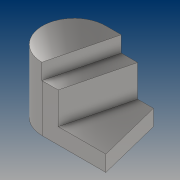
# Autodesk Inventor part: 6
Saved by Autodesk Inventor 2020.2 (Build 242310000, 310)
## iProperties
Created: 2020-09-17
Part Number: 6
Material: 鋼、碳鋼
Document SubType Name: Modeling
Designer: user
Density: 7.85 g/cm^3
Appearance: 半拋光
Mass: 416.126 g
Surface Area: 96.1298 cm^2
Volume: 53.0096 cm^3
Author: user
Autodesk Inventor part; units mm, degrees
ref_plane "YZ Plane" through (0, 0, 0) normal (1, 0, 0) x (0, 1, 0)
ref_plane "XZ Plane" through (0, 0, 0) normal (0, 1, 0) x (-1, 0, 0)
ref_plane "XY Plane" through (0, 0, 0) normal (0, 0, 1) x (1, 0, 0)
sketch "草圖1" plane through (0, 0, 0) normal (0, 1, 0) x (-1, 0, 0)
  circle A0 centre (0, 0) radius 20
  line L0 (0, -20) -> (-40, -20)
  line L1 (-40, -20) -> (-40, 20)
  line L2 (-40, 20) -> (0, 20)
  line L3 (0, 20) -> (0, -20)
  point P0 (0, 20)
  dimension "d0" = 40
  dimension "d1" = 40
  constraints: 8 end point, 3 horizontal, 2 parallel, 1 coincident, 1 perpendicular, 3 other
  measures "d1" distance of L0.start L0.end
extrude "擠出1" add sketch "草圖1" along normal blind 40
sketch "草圖2" plane through (0, 40, 0) normal (0, 1, 0) x (1, 0, 0)
  line L0 (0, 20) -> (40, 20) projected
  line L1 (40, 20) -> (40, -20) projected
  line L2 (40, -20) -> (0, -20) projected
  arc A0 (0, 20) -> (0, -20) centre (0, 0) ccw projected
  line L3 (0, -20) -> (40, -20) projected
  line L4 (40, -20) -> (30, 20)
  dimension "d4" = 10
  constraints: 2 end point, 1 point on line
  measures "d4" distance from line of L4.end L1
extrude "擠出2" cut sketch "草圖2" against normal through all contours L0 L1 L4
sketch "草圖3" plane through (0, 40, 0) normal (0, 1, 0) x (1, 0, 0)
  line L0 (30, 20) -> (0, 20) projected
  line L1 (20, 20) -> (10, -20)
  line L2 (0, -20) -> (40, -20) projected
  line L3 (30, 20) -> (40, -20) projected
  line L4 (40, -20) -> (0, -20) projected
  arc A0 (0, 20) -> (0, -20) centre (0, 0) ccw projected
  line L5 (0, 20) -> (30, 20) projected
  dimension "d7" = 10
  dimension "d8" = 30
  constraints: 2 end point, 2 point on line
  measures "d7" distance of L0.start L1.start
  measures "d8" distance of L2.end L1.end
extrude "擠出3" cut sketch "草圖3" against normal blind 30 contours L3 L2 L1 L0
sketch "草圖4" plane through (0, 40, 0) normal (0, 1, 0) x (1, 0, 0)
  line L0 (20, 20) -> (10, -20) projected
  line L1 (10, -20) -> (0, -20) projected
  arc A0 (0, 20) -> (0, -20) centre (0, 0) ccw projected
  line L2 (0, 20) -> (20, 20) projected
  line L3 (20, 20) -> (0, 20) projected
  line L4 (9.6922, 20) -> (-0.3072, -19.9976)
  line L5 (0, -20) -> (40, -20) projected
  line L6 (10, -20) -> (20, 20) projected
  dimension "d11" = 10
  constraints: 2 end point, 1 parallel, 1 point on circle, 1 point on line
  measures "d11" distance between parallel lines of L0 L4
extrude "擠出4" cut sketch "草圖4" against normal blind 10 contours L0 L1 A0 L4 L2
